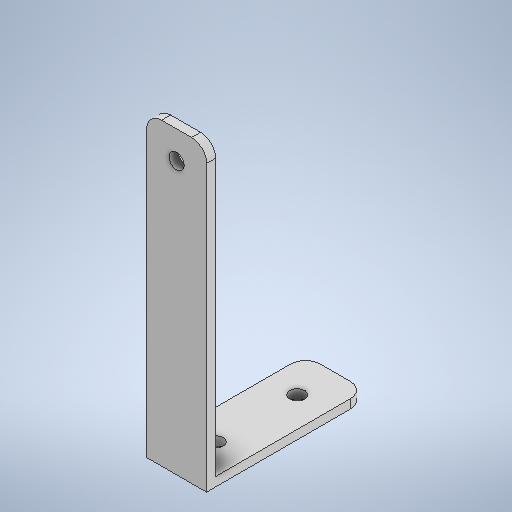
# Autodesk Inventor part: support bar
Saved by Autodesk Inventor 2025.1 (Build 291241020, 241B)
## iProperties
Created: 2025-01-20
Part Number: support bar
Material: Generic
Document SubType Name: Modeling
Designer: User
Density: 1 g/cm^3
Appearance: Default
Author: User
Autodesk Inventor part; units mm, degrees
ref_plane "YZ Plane" through (0, 0, 0) normal (1, 0, 0) x (0, 1, 0)
ref_plane "XZ Plane" through (0, 0, 0) normal (0, 1, 0) x (-1, 0, 0)
ref_plane "XY Plane" through (0, 0, 0) normal (0, 0, 1) x (1, 0, 0)
sketch "Sketch1" plane through (0, 0, 0) normal (0, 1, 0) x (-1, 0, 0)
  line L0 (0, 0) -> (-20, 0)
  line L1 (-20, 0) -> (-20, -50)
  line L2 (-20, -50) -> (0, -50)
  line L3 (0, -50) -> (0, 0)
  circle A0 centre (-10, -10.0524) radius 2.5
  circle A1 centre (-10, -37.2673) radius 2.5
  dimension "d0" = 20
  dimension "d1" = 50
  dimension "d2" = 5
  dimension "d3" = 5
  constraints: 8 end point, 2 centre point, 2 parallel, 1 horizontal, 1 perpendicular
  measures "d0" distance of L2.end L1.end
  measures "d1" distance of L2.end L0.start
  measures "d2" diameter of A0
  measures "d3" diameter of A1
extrude "Extrusion1" add sketch "Sketch1" along normal blind 3
sketch "Sketch2" plane through (0, 0, 0) normal (0, 0, 1) x (1, 0, 0)
  line L0 (0, 0) -> (20, 0)
  line L1 (20, 0) -> (20, 100)
  line L2 (20, 100) -> (0, 100)
  line L3 (0, 100) -> (0, 0)
  circle A0 centre (10, 90.706) radius 2.55
  dimension "d6" = 20
  dimension "d7" = 100
  dimension "d8" = 5.1
  dimension "d9" = 90.706
  constraints: 8 end point, 2 parallel, 1 centre point, 1 horizontal, 1 perpendicular
  measures "d6" distance of L2.end L1.end
  measures "d7" distance of L0.end L1.end
  measures "d8" diameter of A0
  measures "d9" distance from line of L0 A0.centre
extrude "Extrusion2" add sketch "Sketch2" along normal blind 3
fillet "Fillet1" radius 5 2 edges at (20, 1.5, -50) (0, 1.5, -50)
fillet "Fillet2" radius 5 2 edges at (20, 100, 1.5) (0, 100, 1.5)
body "Solid1"
